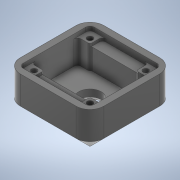
# Autodesk Inventor part: Camera_cover_e-CAM50_CUNX
Saved by Autodesk Inventor 2020 (Build 240168000, 168)
## iProperties
Part Number: Camera_cover_e-CAM50_CUNX
Material: PC/ABS プラスチック
Document SubType Name: Modeling
Designer: Masato Kubotera
Density: 0.357273 g/cm^3
Appearance: 滑らか - 黒
Mass: 20.4693 g
Surface Area: 162.772 cm^2
Volume: 57.2933 cm^3
Description: PLA
Author: Masato Kubotera
Autodesk Inventor part; units mm, degrees
ref_plane "YZ Plane" through (0, 0, 0) normal (1, 0, 0) x (0, 1, 0)
ref_plane "XZ Plane" through (0, 0, 0) normal (0, 1, 0) x (-1, 0, 0)
ref_plane "XY Plane" through (0, 0, 0) normal (0, 0, 1) x (1, 0, 0)
derived "Camera_root_frame_e-CAM50_CUNX.ipt"
sketch "スケッチ1" plane through (0, 0, 0) normal (0, 0, 1) x (1, 0, 0)
  line L0 (15, 15) -> (-15, 15) construction
  line L1 (-15, 15) -> (-15, -15) construction
  line L2 (-15, -15) -> (15, -15) construction
  line L3 (15, -15) -> (15, 15) construction
  line L4 (15, 15) -> (-15, -15) construction
  line L5 (-15, 15) -> (15, -15) construction
  line L6 (-13.14, 13.14) -> (13.14, 13.14) construction
  line L7 (13.14, 13.14) -> (13.14, -13.14) construction
  line L8 (13.14, -13.14) -> (-13.14, -13.14) construction
  line L9 (-13.14, -13.14) -> (-13.14, 13.14) construction
  line L10 (-13.14, 13.14) -> (13.14, -13.14) construction
  line L11 (13.14, 13.14) -> (-13.14, -13.14) construction
  circle A0 centre (-13.14, -13.14) radius 1.1 construction
  line L12 (-15, 0) -> (15, 0) construction
  line L13 (0, 15) -> (0, -15) construction
  circle A1 centre (-13.14, 13.14) radius 1.1 construction
  circle A2 centre (13.14, -13.14) radius 1.1 construction
  circle A3 centre (13.14, 13.14) radius 1.1 construction
  circle A4 centre (-13.14, -13.14) radius 2 construction
  circle A5 centre (-13.14, 13.14) radius 2 construction
  circle A6 centre (13.14, -13.14) radius 2 construction
  circle A7 centre (13.14, 13.14) radius 2 construction
  circle A8 centre (0, 0) radius 7 construction
  circle A9 centre (-5.5, -9) radius 2 construction
  line L14 (-7, 8) -> (7, 8)
  line L15 (8, 7) -> (8, -7)
  line L16 (7, -8) -> (-7, -8)
  line L17 (-8, -7) -> (-8, 7)
  line L18 (-8, 8) -> (8, -8) construction
  line L19 (8, 8) -> (-8, -8) construction
  arc A10 (-7, 8) -> (-8, 7) centre (-7, 7) ccw
  arc A11 (-8, -7) -> (-7, -8) centre (-7, -7) ccw
  arc A12 (7, -8) -> (8, -7) centre (7, -7) ccw
  arc A13 (8, 7) -> (7, 8) centre (7, 7) ccw
  arc A14 (-10, 2) -> (-10, -2) centre (-10, 0) ccw
  line L20 (-10, 2) -> (-8, 2)
  line L21 (-10, -2) -> (-8, -2)
  arc A15 (10, -2) -> (10, 2) centre (10, 0) ccw
  line L22 (10, 2) -> (8, 2)
  line L23 (10, -2) -> (8, -2)
sketch "スケッチ2" plane through (0, 0, 0) normal (0, 0, 1) x (1, 0, 0)
  line L0 (-22.5, 25) -> (22.5, 25)
  line L1 (25, 22.5) -> (25, -22.5)
  line L2 (22.5, -25) -> (-22.5, -25)
  line L3 (-25, -22.5) -> (-25, 22.5)
  line L4 (-25, 25) -> (25, -25) construction
  line L5 (25, 25) -> (-25, -25) construction
  arc A0 (-22.5, 25) -> (-25, 22.5) centre (-22.5, 22.5) ccw
  arc A1 (-25, -22.5) -> (-22.5, -25) centre (-22.5, -22.5) ccw
  arc A2 (22.5, -25) -> (25, -22.5) centre (22.5, -22.5) ccw
  arc A3 (25, 22.5) -> (22.5, 25) centre (22.5, 22.5) ccw
  line L6 (-25, -22.5) -> (25, -22.5) construction
  line L7 (25, -22.5) -> (25, -17.5)
  line L8 (25, -17.5) -> (-25, -17.5) construction
  line L9 (-25, -17.5) -> (-25, -22.5) construction
  line L10 (-25, -22.5) -> (25, -17.5) construction
  line L11 (25, -22.5) -> (-25, -17.5) construction
  line L12 (-25, -20) -> (25, -20) construction
  line L13 (0, 15) -> (0, -15) construction
  circle A4 centre (-20, -20) radius 1.6
  circle A5 centre (20, -20) radius 1.6
  line L14 (-15, 0) -> (15, 0) construction
  circle A6 centre (-20, 20) radius 1.6
  circle A7 centre (20, 20) radius 1.6
  circle A8 centre (-5.5, -9) radius 2 construction
  circle A9 centre (13.14, 13.14) radius 1.1
  circle A10 centre (13.14, -13.14) radius 1.1
  circle A11 centre (-13.14, -13.14) radius 1.1
  circle A12 centre (-13.14, 13.14) radius 1.1
  circle A13 centre (-13.14, -13.14) radius 1.55
  circle A14 centre (13.14, -13.14) radius 1.55
  circle A15 centre (13.14, 13.14) radius 1.55
  circle A16 centre (-13.14, 13.14) radius 1.55
  line L15 (-15, -15) -> (15, -15)
  line L16 (-15, 15) -> (-15, -15)
  line L17 (-15, -7.8919) -> (-15, 0)
  line L18 (0, -15) -> (-7.8919, -15)
  arc A17 (-9.8912, -13.0533) -> (-13.0533, -9.8912) centre (-13.14, -13.14) ccw
  arc A18 (-9.8912, -13.0533) -> (-7.8919, -15) centre (-7.8919, -13) ccw
  arc A19 (-15, -7.8919) -> (-13.0533, -9.8912) centre (-13, -7.8919) ccw
  arc A20 (-13.0533, 9.8912) -> (-15, 7.8919) centre (-13, 7.8919) ccw
  arc A21 (-7.8919, 15) -> (-9.8912, 13.0533) centre (-7.8919, 13) ccw
  line L19 (-15, 7.8919) -> (-15, 0)
  line L20 (0, 15) -> (-7.8919, 15)
  arc A22 (-13.0533, 9.8912) -> (-9.8912, 13.0533) centre (-13.14, 13.14) ccw
  arc A23 (13.0533, -9.8912) -> (15, -7.8919) centre (13, -7.8919) ccw
  arc A24 (7.8919, -15) -> (9.8912, -13.0533) centre (7.8919, -13) ccw
  arc A25 (13.0533, -9.8912) -> (9.8912, -13.0533) centre (13.14, -13.14) ccw
  line L21 (15, -7.8919) -> (15, 0)
  line L22 (15, 7.8919) -> (15, 0)
  arc A26 (15, 7.8919) -> (13.0533, 9.8912) centre (13, 7.8919) ccw
  arc A27 (9.8912, 13.0533) -> (13.0533, 9.8912) centre (13.14, 13.14) ccw
  arc A28 (9.8912, 13.0533) -> (7.8919, 15) centre (7.8919, 13) ccw
  line L23 (0, 15) -> (7.8919, 15)
  line L24 (0, -15) -> (7.8919, -15)
  line L25 (-7.5, -22.5) -> (7.5, -22.5) construction
  line L26 (7.5, -22.5) -> (7.5, -17.5) construction
  line L27 (7.5, -17.5) -> (-7.5, -17.5) construction
  line L28 (-7.5, -17.5) -> (-7.5, -22.5) construction
  line L29 (-7.5, -22.5) -> (7.5, -17.5) construction
  line L30 (7.5, -22.5) -> (-7.5, -17.5) construction
  line L31 (-6.0651, -22.55) -> (6.0651, -22.55)
  line L32 (6.0651, -17.45) -> (-6.0651, -17.45)
  arc A29 (-7.55, -21.0651) -> (-6.0651, -22.55) centre (-6.8075, -21.8075) ccw
  arc A30 (-6.0651, -17.45) -> (-7.55, -18.9349) centre (-6.8075, -18.1925) ccw
  arc A31 (7.55, -18.9349) -> (6.0651, -17.45) centre (6.8075, -18.1925) ccw
  arc A32 (6.0651, -22.55) -> (7.55, -21.0651) centre (6.8075, -21.8075) ccw
  line L33 (-7.55, -22.5) -> (-7.55, -22.55)
  line L34 (-7.55, -18.9349) -> (-7.55, -21.0651)
  line L35 (7.55, -21.0651) -> (7.55, -18.9349)
  arc A33 (-6.0651, 22.55) -> (-7.55, 21.0651) centre (-6.8075, 21.8075) ccw
  line L36 (-7.55, 18.9349) -> (-7.55, 21.0651)
  arc A34 (-7.55, 18.9349) -> (-6.0651, 17.45) centre (-6.8075, 18.1925) ccw
  line L37 (6.0651, 17.45) -> (-6.0651, 17.45)
  line L38 (-6.0651, 22.55) -> (6.0651, 22.55)
  line L39 (7.55, 21.0651) -> (7.55, 18.9349)
  arc A35 (6.0651, 17.45) -> (7.55, 18.9349) centre (6.8075, 18.1925) ccw
  arc A36 (7.55, 21.0651) -> (6.0651, 22.55) centre (6.8075, 21.8075) ccw
  arc A37 (-16, -18) -> (-18, -16) centre (-18, -18) ccw
  line L40 (-16, -18) -> (-16, -23)
  arc A38 (-15.9998, -22.9729) -> (-14, -25) centre (-14, -23) ccw
  line L41 (-16, 18) -> (-16, 23)
  arc A39 (-14, 25) -> (-15.9998, 22.9729) centre (-14, 23) ccw
  arc A40 (15.9998, 22.9729) -> (14, 25) centre (14, 23) ccw
  line L42 (16, 18) -> (16, 23)
  line L43 (16, -18) -> (16, -23)
  arc A41 (14, -25) -> (15.9998, -22.9729) centre (14, -23) ccw
  line L44 (15, 0) -> (-15, 0) construction
  arc A42 (-25, -14) -> (-23, -16) centre (-23, -14) ccw
  line L45 (-23, -16) -> (-18, -16)
  arc A43 (-23, 16) -> (-25, 14) centre (-23, 14) ccw
  line L46 (-23, 16) -> (-18, 16)
  arc A44 (-18, 16) -> (-16, 18) centre (-18, 18) ccw
  arc A45 (16, 18) -> (18, 16) centre (18, 18) ccw
  line L47 (23, 16) -> (18, 16)
  arc A46 (25, 14) -> (23, 16) centre (23, 14) ccw
  arc A47 (23, -16) -> (25, -14) centre (23, -14) ccw
  line L48 (23, -16) -> (18, -16)
  arc A48 (18, -16) -> (16, -18) centre (18, -18) ccw
  point P0 (0, 0)
  point P1 (0, -20)
  point P2 (0, -20)
  point P3 (-10.4749, -15)
  point P4 (-16.5858, -16.5858)
sketch "スケッチ3" plane through (0, 0, 0) normal (0, 0, 1) x (1, 0, 0)
  arc A0 (-25, -22.5) -> (-22.5, -25) centre (-22.5, -22.5) ccw construction
  line L0 (22.5, -25) -> (-22.5, -25) construction
  circle A1 centre (-20, -20) radius 1.6 construction
  line L1 (-25, -22.5) -> (-25, 22.5) construction
  line L2 (-16, -18) -> (-16, -23) construction
  arc A2 (-15.9998, -22.9729) -> (-14, -25) centre (-14, -23) ccw construction
  arc A3 (-25.5, -22.5) -> (-22.5, -25.5) centre (-22.5, -22.5) ccw
  line L3 (-22.5, -25.5) -> (0, -25.5)
  line L4 (-25.5, -22.5) -> (-25.5, 0)
  line L5 (0, 15) -> (0, -15) construction
  line L6 (-15, 0) -> (15, 0) construction
  arc A4 (-16, -18) -> (-16.5858, -16.5858) centre (-18, -18) ccw construction
  line L7 (25, 25) -> (-25, -25) construction
  arc A5 (-16.5, -18) -> (-16.9393, -16.9393) centre (-18, -18) ccw
  line L8 (-16.5, -18) -> (-16.5, -23)
  arc A6 (-16.5, -23) -> (-14, -25.5) centre (-14, -23) ccw
  circle A7 centre (-20, -20) radius 2
  circle A8 centre (0, 0) radius 8
  circle A9 centre (0, 0) radius 7 construction
  arc A10 (-16.9393, -16.9393) -> (-18, -16.5) centre (-18, -18) ccw
  line L9 (-18, -16.5) -> (-23, -16.5)
  arc A11 (-25.5, -14) -> (-23, -16.5) centre (-23, -14) ccw
  line L10 (-20, -30) -> (20, -30)
  line L11 (30, -20) -> (30, 20)
  line L12 (20, 30) -> (-20, 30)
  line L13 (-30, 20) -> (-30, -20)
  line L14 (-30, -30) -> (30, 30) construction
  line L15 (30, -30) -> (-30, 30) construction
  arc A12 (-30, -20) -> (-20, -30) centre (-20, -20) ccw
  arc A13 (20, -30) -> (30, -20) centre (20, -20) ccw
  arc A14 (30, 20) -> (20, 30) centre (20, 20) ccw
  arc A15 (-20, 30) -> (-30, 20) centre (-20, 20) ccw
  arc A16 (-22.5, 25.5) -> (-25.5, 22.5) centre (-22.5, 22.5) ccw
  line L16 (-22.5, 25.5) -> (0, 25.5)
  line L17 (-25.5, 22.5) -> (-25.5, 0)
  arc A17 (-16.9393, 16.9393) -> (-16.5, 18) centre (-18, 18) ccw
  line L18 (-16.5, 18) -> (-16.5, 23)
  arc A18 (-14, 25.5) -> (-16.5, 23) centre (-14, 23) ccw
  circle A19 centre (-20, 20) radius 2
  arc A20 (-18, 16.5) -> (-16.9393, 16.9393) centre (-18, 18) ccw
  line L19 (-18, 16.5) -> (-23, 16.5)
  arc A21 (-23, 16.5) -> (-25.5, 14) centre (-23, 14) ccw
  arc A22 (22.5, -25.5) -> (25.5, -22.5) centre (22.5, -22.5) ccw
  line L20 (22.5, -25.5) -> (0, -25.5)
  line L21 (25.5, -22.5) -> (25.5, 0)
  arc A23 (16.9393, -16.9393) -> (16.5, -18) centre (18, -18) ccw
  line L22 (16.5, -18) -> (16.5, -23)
  arc A24 (14, -25.5) -> (16.5, -23) centre (14, -23) ccw
  circle A25 centre (20, -20) radius 2
  arc A26 (18, -16.5) -> (16.9393, -16.9393) centre (18, -18) ccw
  line L23 (18, -16.5) -> (23, -16.5)
  arc A27 (23, -16.5) -> (25.5, -14) centre (23, -14) ccw
  arc A28 (25.5, 22.5) -> (22.5, 25.5) centre (22.5, 22.5) ccw
  line L24 (22.5, 25.5) -> (0, 25.5)
  arc A29 (16.5, 23) -> (14, 25.5) centre (14, 23) ccw
  line L25 (16.5, 18) -> (16.5, 23)
  arc A30 (16.5, 18) -> (16.9393, 16.9393) centre (18, 18) ccw
  line L26 (18, 16.5) -> (23, 16.5)
  arc A31 (16.9393, 16.9393) -> (18, 16.5) centre (18, 18) ccw
  line L27 (25.5, 22.5) -> (25.5, 0)
  arc A32 (25.5, 14) -> (23, 16.5) centre (23, 14) ccw
  circle A33 centre (20, 20) radius 2
  line L28 (-15.5251, -17.5251) -> (15.5251, -17.5251)
  line L29 (17.5251, -15.5251) -> (17.5251, 15.5251)
  line L30 (15.5251, 17.5251) -> (-15.5251, 17.5251)
  line L31 (-17.5251, 15.5251) -> (-17.5251, -15.5251)
  line L32 (-17.5251, -17.5251) -> (17.5251, 17.5251) construction
  line L33 (17.5251, -17.5251) -> (-17.5251, 17.5251) construction
  arc A34 (-17.5251, -15.5251) -> (-15.5251, -17.5251) centre (-15.5251, -15.5251) ccw
  arc A35 (15.5251, -17.5251) -> (17.5251, -15.5251) centre (15.5251, -15.5251) ccw
  arc A36 (17.5251, 15.5251) -> (15.5251, 17.5251) centre (15.5251, 15.5251) ccw
  arc A37 (-15.5251, 17.5251) -> (-17.5251, 15.5251) centre (-15.5251, 15.5251) ccw
  point P0 (25.5, -14)
  point P1 (25.5, 14)
  point P2 (-25.5, 14)
  point P3 (-25.5, -14)
  point P4 (16.9393, 16.9393)
  point P5 (16.9393, -16.9393)
  point P6 (-16.9393, 16.9393)
  point P7 (16.9393, 16.9393)
  point P8 (16.9393, -16.9393)
  point P9 (-16.9393, -16.9393)
  dimension "d1" = 0.5
  dimension "d2" = 4
  dimension "d3" = 1
  dimension "d4" = 60
  dimension "d5" = 10
  dimension "d14" = 2
  constraints: 56 end point, 56 point on circle, 48 symmetric about line, 33 centre point, 25 point on line, 22 tangent, 6 equal radius, 6 parallel, 5 coincident, 4 midpoint, 3 horizontal, 2 perpendicular, 20 other
  measures "d1" radial gap between concentric circles of A3 A0
  measures "d2" diameter of A7
  measures "d3" radial gap between concentric circles of A8 A9
  measures "d4" distance of L15.end L14.start
  measures "d5" radius of A12
  measures "d14" radius of A34
extrude "押し出し1" add sketch "スケッチ3" against normal blind 30 contours L4 A11 L9 A10 A5 L8 A6 L3 A3 | L4 L17 A21 L19 A20 A37 L31 A34 A10 L9 A11 | A6 L8 A5 A34 L28 A35 A23 L22 A24 L20 L3 | L17 A16 L16 A18 L18 A17 A20 L19 A21 | A24 L22 A23 A26 L23 A27 L21 A22 L20 | A34 L31 A37 L30 A36 L29 A35 L28 | L16 L24 A29 L25 A30 A36 L30 A37 A17 L18 A18 | A27 L23 A26 A35 L29 A36 A31 L26 A32 L27 L21 | L24 A28 L27 A32 L26 A31 A30 L25 A29 | A7 | A12 L13 A15 L12 A14 L11 A13 L10 | A19 | A25 | A33
extrude "押し出し2" cut sketch "スケッチ3" against normal blind 5 contours L4 L17 A21 L19 A20 A37 L31 A34 A10 L9 A11 | A6 L8 A5 A34 L28 A35 A23 L22 A24 L20 L3 | A34 L31 A37 L30 A36 L29 A35 L28 | L16 L24 A29 L25 A30 A36 L30 A37 A17 L18 A18 | A27 L23 A26 A35 L29 A36 A31 L26 A32 L27 L21
extrude "押し出し3" cut sketch "スケッチ3" against normal blind 3 contours L4 A11 L9 A10 A5 L8 A6 L3 A3 | L17 A16 L16 A18 L18 A17 A20 L19 A21 | A24 L22 A23 A26 L23 A27 L21 A22 L20 | L24 A28 L27 A32 L26 A31 A30 L25 A29
extrude "押し出し4" cut sketch "スケッチ3" against normal blind 8 contours A7 | A19 | A25 | A33
extrude "押し出し5" cut sketch "スケッチ3" against normal blind 20 contours A6 L8 A5 A34 L28 A35 A23 L22 A24 L20 L3 | A34 L31 A37 L30 A36 L29 A35 L28 | L16 L24 A29 L25 A30 A36 L30 A37 A17 L18 A18
chamfer "面取り1" distance 10 angle 45 8 edges at (30, 0, -30) (27.0711, -27.0711, -30) (0, -30, -30) (-27.0711, -27.0711, -30) (-30, 0, -30) (-27.0711, 27.0711, -30) (0, 30, -30) (27.0711, 27.0711, -30)
chamfer "面取り2" distance 5 angle 45 1 edges at (-8, 0, -30)
